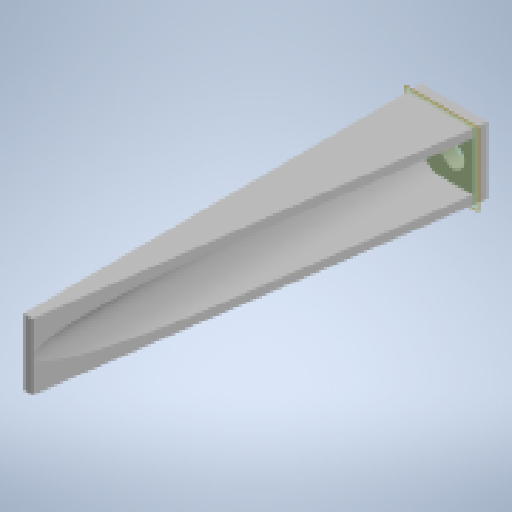
# Autodesk Inventor part: Cable_Chain_Holder
Saved by Autodesk Inventor 2023 (Build 270158000, 158)
## iProperties
Created: 2023-04-30
Part Number: Cable_Chain_Holder
Material: Generic
Document SubType Name: Modeling
Designer: plebbb
Density: 1 g/cm^3
Appearance: Default
Author: plebbb
Autodesk Inventor part; units mm, degrees
ref_plane "YZ Plane" through (0, 0, 0) normal (1, 0, 0) x (0, 1, 0)
ref_plane "XZ Plane" through (0, 0, 0) normal (0, 1, 0) x (-1, 0, 0)
sketch "Sketch1" plane through (0, 0, 0) normal (0, 1, 0) x (-1, 0, 0)
  line L0 (0, 0) -> (17.5, 0)
  line L1 (17.5, 0) -> (17.5, 90)
  line L2 (15.5, 90) -> (17.5, 90)
  line L3 (0, 0) -> (15.5, 90)
  dimension "d0" = 90
  dimension "d1" = 17.5
  dimension "d2" = 2
  constraints: 8 end point, 2 horizontal, 1 perpendicular
  measures "d0" distance of L0.end L1.end
  measures "d1" distance of L0.start L0.end
  measures "d2" distance of L2.start L1.end
extrude "Extrusion1" add sketch "Sketch1" along normal blind 15
ref_plane "Work Plane1" through (0, 0, 3) normal (0, 0, -1) x (-1, 0, 0)
sketch "Sketch2" plane through (0, 0, 3) normal (0, 0, -1) x (-1, 0, 0)
  line L0 (0, 13) -> (10, 13)
  arc A0 (10, 2) -> (10, 13) centre (10, 7.5) ccw
  line L1 (10, 2) -> (0, 2)
  line L2 (0, 15) -> (0, 13)
  line L3 (0, 2) -> (0, 0)
  line L4 (0, 15) -> (17.5, 15)
  line L5 (0, 0) -> (17.5, 0) projected
  line L6 (17.5, 15) -> (17.5, 0)
  line L7 (17.5, 0) -> (0, 0)
  line L8 (15.5, 7.5) -> (17.5, 7.5) construction
  line L9 (17.5, 0) -> (17.5, 15) construction
  line L10 (0, 2) -> (0, 13)
  line L11 (0, 0) -> (0, 15) projected
  dimension "d5" = 2
  constraints: 18 end point, 3 horizontal, 3 point on circle, 2 collinear, 2 equal length, 2 perpendicular, 2 tangent, 1 centre point, 1 midpoint, 1 vertical
  measures "d5" distance of L8.start L8.end
extrude "Extrusion2" cut sketch "Sketch2" against normal up to surface (87 mm away) contours L0 A0 L1 L10
sketch "Sketch3" plane through (0, 0, 0) normal (0, 0, -1) x (-1, 0, 0)
  circle A0 centre (5, 7.5) radius 2.613
  line L0 (5, 7.5) -> (0, 7.5) construction
  line L1 (0, 0) -> (0, 15) projected
  dimension "d9" = 5.226
  dimension "d10" = 5
  constraints: 2 end point, 1 centre point, 1 horizontal, 1 midpoint
  measures "d9" diameter of A0
  measures "d10" distance of L0.start L0.end
extrude "Extrusion3" cut sketch "Sketch3" against normal blind 10
fillet "Fillet1" radius 2 2 edges at (-17.5, 0, 45) (-17.5, 15, 45)
body "Solid1"
